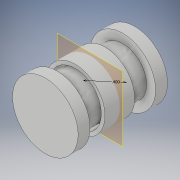
# Autodesk Inventor part: Ring Tolerance Test 6
Saved by Autodesk Inventor 2018 (Build 220112000, 112)
## iProperties
Created: 2019-08-26
Part Number: Ring Tolerance Test 6
Material: Generic
Document SubType Name: Modeling
Designer: 871357
Density: 1 g/cm^3
Appearance: Default
Author: 871357
Autodesk Inventor part; units mm, degrees
ref_plane "YZ Plane" through (0, 0, 0) normal (1, 0, 0) x (0, 1, 0)
ref_plane "XZ Plane" through (0, 0, 0) normal (0, 1, 0) x (-1, 0, 0)
sketch "Sketch1" plane through (0, 0, 0) normal (0, 0, 1) x (1, 0, 0)
  circle A0 centre (0, 0) radius 5.08
  dimension "d0" = 10.16
  constraints: 1 centre point, 1 coincident
  measures "d0" diameter of A0
extrude "Extrusion1" add sketch "Sketch1" along normal blind 10.16
ref_plane "Work Plane1" through (0, 0, 5.08) normal (0, 0, -1) x (-1, 0, 0)
sketch "Sketch4" plane through (0, 0, 0) normal (0, 0, -1) x (-1, 0, 0)
  circle A0 centre (0, 0) radius 5.588
  circle A1 centre (0, 0) radius 6.35
  dimension "d13" = 11.176
  dimension "d14" = 12.7
  constraints: 2 centre point, 2 coincident
  measures "d13" diameter of A0
  measures "d14" diameter of A1
extrude "Extrusion4" add sketch "Sketch4" against normal blind 6.35
extrude "Extrusion5" add sketch "Sketch1" against normal blind 3.81
sketch "Sketch5" plane through (0, 0, -3.81) normal (0, 0, -1) x (-1, 0, 0)
  circle A0 centre (0, 0) radius 6.985
  dimension "d25" = 13.97
  constraints: 1 centre point, 1 coincident
  measures "d25" diameter of A0
extrude "Extrusion6" add sketch "Sketch5" along normal blind 2.54
ref_plane "Work Plane2" through (0, 0, 3.175) normal (0, 0, 1) x (1, 0, 0)
mirror "Mirror2" about plane through (0, 0, 3.175) normal (0, 0, 1) of "Extrusion6"
body "Solid1"
